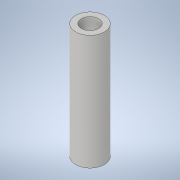
# Autodesk Inventor part: 30_Cube_Z_Focus_MGN_NEMA_Motorcoupling_Captive_v3
Saved by Autodesk Inventor 2022 (Build 260153000, 153)
## iProperties
Created: 2021-04-26
Part Number: 30_Cube_Z_Focus_MGN_NEMA_Motorcoupling_Captive_v3
Material: Generic
Document SubType Name: Modeling
Designer: diederichbenedict
Density: 1 g/cm^3
Appearance: Default
Mass: 1.15069 g
Surface Area: 11.4691 cm^2
Volume: 1.15069 cm^3
Author: diederichbenedict
Autodesk Inventor part; units mm, degrees
ref_plane "YZ Plane" through (0, 0, 0) normal (1, 0, 0) x (0, 1, 0)
ref_plane "XZ Plane" through (0, 0, 0) normal (0, 1, 0) x (-1, 0, 0)
ref_plane "XY Plane" through (0, 0, 0) normal (0, 0, 1) x (1, 0, 0)
sketch "Sketch8" plane through (0, 0, 0) normal (0, 1, 0) x (-1, 0, 0)
  circle A0 centre (0, 0) radius 4.25
  line L0 (-1.5588, -2.7) -> (-3.1177, 0)
  line L1 (-3.1177, 0) -> (-1.5588, 2.7)
  line L2 (-1.5588, 2.7) -> (1.5588, 2.7)
  line L3 (1.5588, 2.7) -> (3.1177, 0)
  line L4 (3.1177, 0) -> (1.5588, -2.7)
  line L5 (1.5588, -2.7) -> (-1.5588, -2.7)
  line L6 (-5.95, 0) -> (5.95, 0) projected
  dimension "d57" = 8.5
  dimension "d58" = 5.4
  constraints: 12 end point, 2 coincident, 1 centre point, 1 parallel, 13 other
  measures "d57" diameter of A0
  measures "d58" distance between parallel lines of L5 L2
extrude "Extrusion7" add sketch "Sketch8" along normal blind 4 contours L6 L3 L2 L1 A0 | A0 L6 L0 L5 L4
sketch "Sketch9" plane through (0, 4, 0) normal (0, 1, 0) x (1, 0, 0)
  circle A0 centre (0, 0) radius 4.25 projected
  line L0 (-3.1177, 0) -> (-1.5588, 2.7) projected
  line L1 (-1.5588, 2.7) -> (1.5588, 2.7) projected
  line L2 (1.5588, 2.7) -> (3.1177, 0) projected
  line L3 (3.1177, 0) -> (1.5588, -2.7) projected
  line L4 (1.5588, -2.7) -> (-1.5588, -2.7) projected
  line L5 (-1.5588, -2.7) -> (-3.1177, 0) projected
  circle A1 centre (0, 0) radius 2.55
  dimension "d61" = 5.1
  constraints: 1 centre point
  measures "d61" diameter of A1
extrude "Extrusion8" add sketch "Sketch9" along normal blind 30 contours A0 | L0 L1 L2 L3 L4 L5
body "Solid2"
